Samsungholster (Autodesk Fusion 360 design; units mm, degrees)
Autodesk Fusion 360 part; units mm, degrees
sketch "Sketch1" plane through (0, 0, 0) normal (0, 0, 1) x (1, 0, 0)
  line L0 (38.1, 6.1) -> (-38.1, 6.1)
  line L1 (-40.1, 4.1) -> (-40.1, -4.1)
  line L2 (-38.1, -6.1) -> (38.1, -6.1)
  line L3 (40.1, -4.1) -> (40.1, 4.1)
  line L4 (40.1, 6.1) -> (-40.1, -6.1) construction
  line L5 (-40.1, 6.1) -> (40.1, -6.1) construction
  arc A0 (-38.1, 6.1) -> (-40.1, 4.1) centre (-38.1, 4.1) ccw
  arc A1 (-40.1, -4.1) -> (-38.1, -6.1) centre (-38.1, -4.1) ccw
  arc A2 (40.1, 4.1) -> (38.1, 6.1) centre (38.1, 4.1) ccw
  arc A3 (38.1, -6.1) -> (40.1, -4.1) centre (38.1, -4.1) ccw
  line L6 (-41.9, 4.1) -> (-41.9, -4.1)
  arc A4 (-41.9, -4.1) -> (-38.1, -7.9) centre (-38.1, -4.1) ccw
  line L7 (-38.1, -7.9) -> (38.1, -7.9)
  arc A5 (38.1, -7.9) -> (41.9, -4.1) centre (38.1, -4.1) ccw
  line L8 (41.9, -4.1) -> (41.9, 4.1)
  arc A6 (41.9, 4.1) -> (38.1, 7.9) centre (38.1, 4.1) ccw
  line L9 (38.1, 7.9) -> (-38.1, 7.9)
  arc A7 (-38.1, 7.9) -> (-41.9, 4.1) centre (-38.1, 4.1) ccw
  line L10 (0, 7.9) -> (-30, 7.9)
  line L11 (-30, 7.9) -> (-30, 32.9)
  line L12 (-30, 32.9) -> (0, 32.9)
  line L13 (0, 32.9) -> (0, 7.9)
  line L14 (30, 32.9) -> (0, 32.9)
  line L15 (30, 7.9) -> (30, 32.9)
  line L16 (0, 7.9) -> (30, 7.9)
  line L17 (0, -6.1) -> (0, 6.1)
  arc A8 (-15.2233, 7.9) -> (-15.3767, 7.9) centre (-15.3, 0) ccw
  arc A9 (-20.3205, 6.1) -> (-20.3205, -6.1) centre (-15.3, 0) ccw
  arc A10 (-15.3767, -7.9) -> (-15.2233, -7.9) centre (-15.3, 0) ccw
  arc A11 (-10.2795, -6.1) -> (-10.2795, 6.1) centre (-15.3, 0) ccw
  arc A12 (15.3767, 7.9) -> (15.2233, 7.9) centre (15.3, 0) ccw
  arc A13 (20.3205, -6.1) -> (20.3205, 6.1) centre (15.3, 0) ccw
  arc A14 (10.2795, 6.1) -> (10.2795, -6.1) centre (15.3, 0) ccw
  arc A15 (15.2233, -7.9) -> (15.3767, -7.9) centre (15.3, 0) ccw
  dimension "d1" = 80.2
  dimension "d2" = 12.2
  dimension "d3" = 2
  dimension "d4" = 2
  dimension "d5" = 2
  dimension "d6" = 1.8
  dimension "d17" = 30
  dimension "d18" = 25
  dimension "d65" = 24.8
  constraint horizontal L0
  constraint perpendicular L0 L1
  constraint parallel L0 L2
  constraint parallel L1 L3
  constraint coincident L4 origin
  constraint coincident L5 origin
  constraint coincident L5.start L0
  constraint coincident L5.start L1
  constraint tangent L0 A0
  constraint tangent L1 A0
  constraint coincident L4.end L1
  constraint coincident L4.end L2
  constraint tangent L1 A1
  constraint tangent L2 A1
  constraint coincident L4.start L0
  constraint coincident L4.start L3
  constraint tangent L0 A2
  constraint tangent L3 A2
  constraint equal A1 A2
  constraint coincident L5.end L3
  constraint coincident L5.end L2
  constraint tangent L3 A3
  constraint tangent L2 A3
  constraint horizontal L10
  constraint vertical L11
  constraint horizontal L12
  constraint vertical L13
  constraint midpoint L9 L10.start
  constraint symmetric L10.start L13 L16.start
  constraint symmetric L10.end L13 L15.start
  constraint symmetric L11.end L13 L14.start
  constraint symmetric L12.end L13 L14.end
  constraint midpoint L2 L17.start
  constraint midpoint L0 L17.end
  constraint symmetric L17 A8 A14
  constraint coincident L0 A11.end
  constraint coincident L9 A8.start
  constraint coincident L9 A8.end
  constraint coincident L0 A9.start
  constraint concentric A8 A9
  constraint coincident L2 A9.end
  constraint coincident L7 A10.start
  constraint concentric A9 A10
  constraint coincident L7 A10.end
  constraint coincident L2 A11.start
  constraint concentric A10 A11
  constraint coincident L9 A12.end
  constraint coincident L0 A14.start
  constraint coincident L0 A13.end
  constraint coincident L9 A12.start
  constraint concentric A12 A14
  constraint coincident L7 A15.end
  constraint coincident L2 A13.start
  constraint concentric A13 A14
  constraint coincident L2 A14.end
  constraint coincident L7 A15.start
  constraint concentric A14 A15
  measures "d1" distance of L4.end L5.end
  measures "d2" distance of L5.start L4.end
  measures "d3" radius of A0
  measures "d4" radius of A1
  measures "d5" radius of A3
  measures "d17" distance of L10.start L10.end
  measures "d18" distance of L10.start L12.end
  measures "d65" distance of L1 A8.centre
extrude "Extrude1" add sketch "Sketch1" along normal blind 100 contours L6 A4 L7 A5 L8 A6 L9 A7 L10 L16 A8 A10 A12 A15
extrude "Extrude2" add sketch "Sketch1" against normal blind 2.2 contours L0 L2 L3 A2 A3 A13 | L0 L2 A13 A14 | L0 L2 L17 A14 | L0 L2 L17 A11 | L0 L2 A9 A11 | L0 L1 L2 A0 A1 A9 | L6 A4 L7 A5 L8 A6 L9 A7 L10 L16 A8 A10 A12 A15
sketch "Sketch2" plane through (0, 0, 0) normal (1, 0, 0) x (0, 1, 0)
  line L0 (7.9, -2.2) -> (7.9, 100)
  line L1 (7.9, 79.9745) -> (17.9, 79.9745)
  line L2 (19.9, 77.9745) -> (19.9, 41.9745)
  line L3 (17.9, 39.9745) -> (7.9, 39.9745)
  line L4 (7.9, 39.9745) -> (7.9, 79.9745)
  arc A0 (19.9, 77.9745) -> (17.9, 79.9745) centre (17.9, 77.9745) ccw
  arc A1 (17.9, 39.9745) -> (19.9, 41.9745) centre (17.9, 41.9745) ccw
  arc A2 (24.2106, 77.9745) -> (17.9, 84.2851) centre (17.9, 77.9745) ccw
  line L5 (7.9, 84.2851) -> (17.9, 84.2851)
  line L6 (17.9, 35.6639) -> (7.9, 35.6639)
  arc A3 (17.9, 35.6639) -> (24.2106, 41.9745) centre (17.9, 41.9745) ccw
  line L7 (24.2106, 77.9745) -> (24.2106, 41.9745)
  line L8 (7.9, 79.9745) -> (7.9, 84.2851)
  line L9 (7.9, 39.9745) -> (7.9, 35.6639)
  line L10 (7.9, 99.7641) -> (13.9, 99.7641)
  line L11 (13.9, 99.7641) -> (13.9, 89.7641)
  line L12 (13.9, 89.7641) -> (7.9, 89.7641)
  line L13 (7.9, 89.7641) -> (7.9, 99.7641)
  line L14 (11.9289, 96.4792) -> (9.8711, 93.0491)
  circle A4 centre (10.9, 94.7641) radius 2
  line L15 (0, 100) -> (0, 86.0916)
  line L16 (-7.9, 99.7641) -> (-13.9, 99.7641)
  line L17 (-8.9372, 89.7641) -> (-7.9, 89.7641)
  line L18 (-7.9, 89.7641) -> (-7.9, 99.7641)
  arc A5 (-8.9001, 94.7492) -> (-10.6292, 96.7457) centre (-10.9, 94.7641) ccw
  line L19 (-13.9, 99.8084) -> (-13.9, 99.7641)
  line L20 (-16.1106, 98.0186) -> (-16.1106, 99.7641)
  line L21 (-16.1106, 98.0186) -> (-10.6927, 96.7543)
  line L22 (-13.9, 99.7641) -> (-16.1106, 99.7641)
  line L23 (-8.9001, 94.7492) -> (-8.9372, 89.7641)
  spline S0 degree 5 poles (-10.6927, 96.7543) (-10.6902, 96.7539) (-10.6851, 96.7532) (-10.6775, 96.7522) (-10.6673, 96.7508) (-10.6546, 96.7491) (-10.6445, 96.7478) (-10.6368, 96.7467) (-10.6318, 96.7461) (-10.6292, 96.7457) knots 0 0 0 0 0 0 0.2 0.4 0.6 0.8 1 1 1 1 1 1
  point P0 (19.9, 79.9745)
  dimension "d11" = 12
  dimension "d13" = 2
  dimension "d41" = 6
  dimension "d42" = 10
  dimension "d43" = 4
  constraint horizontal L1
  constraint vertical L2
  constraint horizontal L3
  constraint vertical L4
  constraint coincident L0 L1.start
  constraint coincident P0 L1
  constraint coincident P0 L2
  constraint tangent L1 A0
  constraint tangent L2 A0
  constraint tangent L2 A1
  constraint tangent L3 A1
  constraint equal A0 A1
  constraint coincident L0 L5.start
  constraint coincident L0 L6.end
  constraint concentric A0 A2
  constraint parallel L1 L5
  constraint parallel L3 L6
  constraint concentric A1 A3
  constraint parallel L2 L7
  constraint tangent A2 L7
  constraint tangent L6 A3
  constraint tangent A2 L5
  constraint tangent A3 L7
  constraint horizontal L10
  constraint vertical L11
  constraint horizontal L12
  constraint vertical L13
  constraint coincident L0 L10.start
  constraint coincident A4 L14.start
  constraint coincident L14 A4.centre
  constraint coincident A4 L14.end
  constraint vertical L15
  constraint symmetric L10.start L15 L16.start
  constraint symmetric L10.end L15 L16.end
  constraint symmetric L12.end L15 L17.end
  constraint symmetric A4 L15 A5
  constraint vertical L19
  constraint vertical L20
  constraint perpendicular L20 L22
  constraint tangent A5 L23
  measures "d11" distance of L1.start P0
  measures "d13" radius of A0
  measures "d41" distance of L10.start L10.end
  measures "d42" distance of L10.start L12.end
  measures "d43" diameter of A4
extrude "Extrude4" add sketch "Sketch2" along normal mid plane 74 contours L0 L1 L2 L3 A0 A1 A2 L5 L6 A3 L7 L8 L9
extrude "Extrude5" cut sketch "Sketch1" along normal blind 90 contours L9 L10 L11 L12 L13 A8 | L9 L13 L14 L15 L16 A12
fillet "Fillet1" radius 7.5 4 edges at (30, 7.9, 82.1298) (30, 7.9, 37.8192) (-30, 7.9, 82.1298) (-30, 7.9, 37.8192)
fillet "Fillet2" radius 7.5 6 edges at (29.75, 7.9, 84.2851) (-29.75, 7.9, 84.2851) (29.75, 7.9, 35.6639) (-29.75, 7.9, 84.2851) (-29.75, 7.9, 35.6639) (29.75, 7.9, 35.6639)
fillet "Fillet3" radius 5 6 edges at (-29.75, 7.9, 39.9745) (29.75, 7.9, 39.9745) (-29.75, 7.9, 39.9745) (29.75, 7.9, 79.9745) (-29.75, 7.9, 79.9745) (29.75, 7.9, 79.9745)
sketch "Sketch3" plane through (0, 0, 0) normal (1, 0, 0) x (0, 1, 0)
  line L0 (-4.1, -2.2) -> (-4.1, 100)
  line L1 (-4.1, 100) -> (4.1, 100)
  line L2 (4.1, -2.2) -> (-4.1, -2.2)
  line L3 (4.1, 100) -> (-4.1, 100)
  line L4 (-4.1, 100) -> (-4.1, 80)
  line L5 (-4.1, 80) -> (4.1, 80)
  line L6 (4.1, 80) -> (4.1, 100)
  line L7 (4.1, 100) -> (4.1, 0)
  line L8 (4.1, 0) -> (4.1, -2.2)
  dimension "d32" = 20
  constraint horizontal L3
  constraint vertical L4
  constraint horizontal L5
  constraint vertical L6
  constraint coincident L0 L4.end
  constraint coincident L1.end L3.start
  measures "d32" distance of L3 L5
extrude "Extrude6" cut sketch "Sketch3" along normal mid plane 100 contours L0 L1 L3 L4 L5 L6 L7
fillet "Fillet4" radius 2 1 edges at (-40.1, 0, 80)
fillet "Fillet5" radius 1.5 4 edges at (-41, 4.1, 100) (-41, -4.1, 100) (41, 4.1, 100) (41, -4.1, 100)
fillet "Fillet6" radius 2 1 edges at (40.1, 0, 80)
extrude "Extrude7" add sketch "Sketch2" along normal mid plane 10 contours L0 L10 L11 L12 L13
fillet "Fillet7" radius 5.5 1 edges at (0, 7.9, 89.7641)
fillet "Fillet8" radius 0.5 4 edges at (5, 13.9, 94.7641) (-5, 13.9, 94.7641) (0, 13.9, 89.7641) (0, 13.9, 99.7641)
sketch "Sketch4" plane through (0, 0, 0) normal (1, 0, 0) x (0, 1, 0)
extrude "Extrude10" add sketch "Sketch2" along normal mid plane 10 contours L16 L17 L18 A5 L20 L21 L22 L23 S0
chamfer "Chamfer7" distance 3 angle 45 2 edges at (5, -7.9, 94.7641) (-5, -7.9, 94.7641)
fillet "Fillet14" radius 5.5 1 edges at (0, -7.9, 89.7641)
fillet "Fillet15" radius 1.5 2 edges at (5, -16.1106, 98.8914) (-5, -16.1106, 98.8914)
fillet "Fillet12" radius 1 14 edges at (-41.9, -4.1, 89.25) (-41.8729, -4.5532, 99.5743) (-40.1905, -7.2733, 100) (0, -7.9, 100) (40.1905, -7.2733, 100) (41.8729, -4.5532, 99.5743) (41.9, -4.1, 89.25) (41.9, 4.1, 89.25) (41.8729, 4.5532, 99.5743) (40.1905, 7.2733, 100) (0, 7.9, 100) (-40.1905, 7.2733, 100) (-41.8729, 4.5532, 99.5743) (-41.9, 4.1, 89.25)
fillet "Fillet13" radius 0.5 8 edges at (41.9, 0, -2.2) (40.787, -6.787, -2.2) (0, -7.9, -2.2) (-40.787, -6.787, -2.2) (-41.9, 0, -2.2) (-40.787, 6.787, -2.2) (0, 7.9, -2.2) (40.787, 6.787, -2.2)
extrude "Extrude9" cut sketch "Sketch1" against normal blind 15 contours L0 L2 A13 A14 | L0 L2 A9 A11
